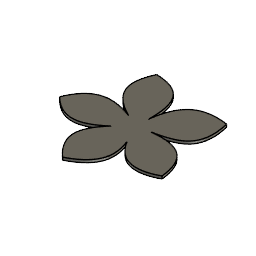
lidwithflowers (Autodesk Fusion 360 archive; units mm, degrees)
design "flower"
part number: 2026-03-09-21-13-14-938
Autodesk Fusion 360 part; units mm, degrees
sketch "Sketch1" plane through (0, 0, 0) normal (0, 0, 1) x (1, 0, 0)
  spline S0 degree 5 poles (0, 0) (-1.4044, 0.5318) (-4.1361, 1.6164) (-8.0024, 3.3065) (-12.6869, 5.6888) (-17.7022, 8.8964) (-21.7919, 12.3572) (-24.8624, 16.0968) (-26.8352, 20.1365) (-27.7054, 24.4779) (-27.5355, 29.1037) (-26.6256, 33.0161) (-25.5341, 36.0622) (-24.6274, 38.1419) (-24.1293, 39.194) knots 0 0 0 0 0 0 0.1 0.2 0.3 0.4 0.5 0.6 0.7 0.8 0.9 1 1 1 1 1 1
  spline S1 degree 5 poles (0, 0) (-1.4044, 0.5318) (-4.1361, 1.6164) (-8.0024, 3.3065) (-12.6869, 5.6888) (-17.7022, 8.8964) (-21.7919, 12.3572) (-24.8624, 16.0968) (-26.8352, 20.1365) (-27.7054, 24.4779) (-27.5355, 29.1037) (-26.6256, 33.0161) (-25.5341, 36.0622) (-24.6274, 38.1419) (-24.1293, 39.194) knots 0 0 0 0 0 0 0.1 0.2 0.3 0.4 0.5 0.6 0.7 0.8 0.9 1 1 1 1 1 1
  spline S2 degree 5 poles (0, 0) (0.161, 1.5019) (0.4296, 4.4479) (0.6723, 8.6935) (0.6692, 13.999) (0.0791, 19.9822) (-1.1604, 25.2356) (-3.1172, 29.6735) (-5.8469, 33.2284) (-9.3505, 35.9027) (-13.5777, 37.7644) (-17.4913, 38.6674) (-20.7044, 39.0444) (-22.9675, 39.1658) (-24.1293, 39.194) knots 0 0 0 0 0 0 0.1 0.2 0.3 0.4 0.5 0.6 0.7 0.8 0.9 1 1 1 1 1 1
  line L0 (-0.8299, -7.7405) -> (0.8299, 7.7405)
  line L1 (-16.8676, 39.0177) -> (-31.3911, 39.3704)
  spline S3 degree 5 poles (0, 0) (-1.3491, 0.6615) (-4.0099, 1.9145) (-7.8889, 3.5841) (-12.8327, 5.3829) (-18.6044, 6.8642) (-23.9261, 7.4959) (-28.7518, 7.1886) (-33.0434, 5.8677) (-36.7985, 3.5283) (-40.0482, 0.2302) (-42.2726, -3.1195) (-43.7428, -6.0066) (-44.6363, -8.0951) (-45.0613, -9.1803) knots 0 0 0 0 0 0 0.1 0.2 0.3 0.4 0.5 0.6 0.7 0.8 0.9 1 1 1 1 1 1
  line L2 (6.9899, -3.4272) -> (-6.9899, 3.4272)
  line L3 (-42.412, -2.4168) -> (-47.7107, -15.9438)
  spline S4 degree 5 poles (0, 0) (-1.3491, 0.6615) (-4.0099, 1.9145) (-7.8889, 3.5841) (-12.8327, 5.3829) (-18.6044, 6.8642) (-23.9261, 7.4959) (-28.7518, 7.1886) (-33.0434, 5.8677) (-36.7985, 3.5283) (-40.0482, 0.2302) (-42.2726, -3.1195) (-43.7428, -6.0066) (-44.6363, -8.0951) (-45.0613, -9.1803) knots 0 0 0 0 0 0 0.1 0.2 0.3 0.4 0.5 0.6 0.7 0.8 0.9 1 1 1 1 1 1
  line L4 (6.9899, -3.4272) -> (-6.9899, 3.4272)
  line L5 (-42.412, -2.4168) -> (-47.7107, -15.9438)
  spline S5 degree 5 poles (0, 0) (-0.9693, -1.1417) (-2.9022, -3.3449) (-5.7844, -6.4087) (-9.5925, -10.0038) (-14.2906, -13.6228) (-18.9201, -16.2785) (-23.4744, -17.8743) (-27.9477, -18.3301) (-32.3398, -17.6432) (-36.6555, -15.8796) (-40.0511, -13.6681) (-42.5677, -11.5861) (-44.2323, -10.0131) (-45.0613, -9.1803) knots 0 0 0 0 0 0 0.1 0.2 0.3 0.4 0.5 0.6 0.7 0.8 0.9 1 1 1 1 1 1
  spline S6 degree 5 poles (0, 0) (0.0283, 1.4963) (0.136, 4.4186) (0.4509, 8.5916) (1.1827, 13.7276) (2.6537, 19.384) (4.7355, 24.2021) (7.4856, 28.1029) (10.9482, 31.0259) (15.115, 32.9823) (19.9411, 34.0338) (24.2903, 34.2048) (27.81, 33.9793) (30.2692, 33.6741) (31.527, 33.4829) knots 0 0 0 0 0 0 0.1 0.2 0.3 0.4 0.5 0.6 0.7 0.8 0.9 1 1 1 1 1 1
  spline S7 degree 5 poles (0, 0) (1.4959, 0.2337) (4.4302, 0.7106) (8.6588, 1.4539) (13.9298, 2.5282) (19.7777, 4.1636) (24.7136, 6.2859) (28.5715, 9.0795) (31.2351, 12.671) (32.7317, 17.0435) (33.2019, 22.0641) (32.8885, 26.4674) (32.3275, 29.9231) (31.8167, 32.2864) (31.527, 33.4829) knots 0 0 0 0 0 0 0.1 0.2 0.3 0.4 0.5 0.6 0.7 0.8 0.9 1 1 1 1 1 1
  line L6 (-7.6915, -1.2018) -> (7.6915, 1.2018)
  line L7 (33.2361, 26.4229) -> (29.8179, 40.5428)
  spline S8 degree 5 poles (0, 0) (1.4535, 0.332) (4.306, 0.9314) (8.4216, 1.6365) (13.5773, 2.1822) (19.4296, 2.1606) (24.6313, 1.3658) (29.12, -0.2764) (32.8467, -2.8242) (35.8172, -6.2706) (38.0787, -10.5597) (39.3621, -14.6158) (40.047, -17.9879) (40.3821, -20.3803) (40.5193, -21.6125) knots 0 0 0 0 0 0 0.1 0.2 0.3 0.4 0.5 0.6 0.7 0.8 0.9 1 1 1 1 1 1
  spline S9 degree 5 poles (0, 0) (0.5946, -1.3429) (1.7894, -3.9529) (3.5989, -7.6402) (6.0586, -12.0947) (9.2832, -16.8423) (12.7487, -20.69) (16.5407, -23.5472) (20.7174, -25.3334) (25.2686, -26.0299) (30.1306, -25.6638) (34.2064, -24.5467) (37.3375, -23.2554) (39.4539, -22.1936) (40.5193, -21.6125) knots 0 0 0 0 0 0 0.1 0.2 0.3 0.4 0.5 0.6 0.7 0.8 0.9 1 1 1 1 1 1
  line L8 (-3.1516, 7.1184) -> (3.1516, -7.1184)
  line L9 (34.1423, -25.0907) -> (46.8964, -18.1344)
  spline S10 degree 5 poles (0, 0) (0.7967, -1.2541) (2.3115, -3.7331) (4.3475, -7.3642) (6.582, -12.0279) (8.5184, -17.5405) (9.5135, -22.7048) (9.4771, -27.4873) (8.3384, -31.8618) (6.1063, -35.8316) (2.8488, -39.4219) (-0.5174, -42.0128) (-3.4436, -43.8074) (-5.5699, -44.9388) (-6.677, -45.4883) knots 0 0 0 0 0 0 0.1 0.2 0.3 0.4 0.5 0.6 0.7 0.8 0.9 1 1 1 1 1 1
  spline S11 degree 5 poles (0, 0) (-1.077, -1.0358) (-3.1694, -3.0841) (-6.1224, -6.087) (-9.6664, -9.9615) (-13.3027, -14.6398) (-15.9606, -19.2129) (-17.4568, -23.7335) (-17.6559, -28.2341) (-16.5671, -32.7078) (-14.3143, -37.1157) (-11.6997, -40.5486) (-9.338, -43.0498) (-7.5925, -44.6814) (-6.677, -45.4883) knots 0 0 0 0 0 0 0.1 0.2 0.3 0.4 0.5 0.6 0.7 0.8 0.9 1 1 1 1 1 1
  line L10 (5.6112, 5.3961) -> (-5.6112, -5.3961)
  line L11 (-12.1265, -40.6854) -> (-1.2275, -50.2912)
  spline S12 degree 5 poles (0, 0) (-1.077, -1.0358) (-3.1694, -3.0841) (-6.1224, -6.087) (-9.6664, -9.9615) (-13.3027, -14.6398) (-15.9606, -19.2129) (-17.4568, -23.7335) (-17.6559, -28.2341) (-16.5671, -32.7078) (-14.3143, -37.1157) (-11.6997, -40.5486) (-9.338, -43.0498) (-7.5925, -44.6814) (-6.677, -45.4883) knots 0 0 0 0 0 0 0.1 0.2 0.3 0.4 0.5 0.6 0.7 0.8 0.9 1 1 1 1 1 1
  line L12 (5.6112, 5.3961) -> (-5.6112, -5.3961)
  line L13 (-12.1265, -40.6854) -> (-1.2275, -50.2912)
  spline S13 degree 5 poles (0, 0) (0.7967, -1.2541) (2.3115, -3.7331) (4.3475, -7.3642) (6.582, -12.0279) (8.5184, -17.5405) (9.5135, -22.7048) (9.4771, -27.4873) (8.3384, -31.8618) (6.1063, -35.8316) (2.8488, -39.4219) (-0.5174, -42.0128) (-3.4436, -43.8074) (-5.5699, -44.9388) (-6.677, -45.4883) knots 0 0 0 0 0 0 0.1 0.2 0.3 0.4 0.5 0.6 0.7 0.8 0.9 1 1 1 1 1 1
  point P0 (-25.6418, 18.0134)
  point P1 (-4.5236, 31.2686)
  point P2 (-25.6418, 18.0134)
  point P3 (-30.6833, 6.4459)
  point P4 (-30.6833, 6.4459)
  point P5 (-25.4504, -17.9323)
  point P6 (-7.2961, 0.1709)
  point P7 (-0.2043, -8.3822)
  point P8 (-0.2043, -8.3822)
  point P9 (5.6112, 5.3961)
  point P10 (8.646, 28.8559)
  point P11 (29.3681, 10.4762)
  point P12 (6.6784, -3.8501)
  point P13 (30.2958, -1.2755)
  point P14 (18, -24)
  point P15 (8.9369, -28.9257)
  point P16 (-17.3527, -25.334)
  point P17 (-1.5601, -7.6131)
  point P18 (8.9369, -28.9257)
  point P19 (-17.3527, -25.334)
extrude "Extrude1" add sketch "Sketch1" along normal blind 1
scale "Scale1" factor 0.2 about (-45.0613, -9.1803, 0) bodies 1
scale "Scale2" factor 0.5 about (-29.7437, -0.6476, 0.2) bodies 1
extrude "Extrude2" add 1 faces at (-32.6421, -4.6736, 0.2) along direction (0, 0, 1) blind 0.09
